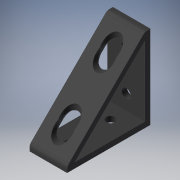
# Autodesk Inventor part: 30-4336 Aluminum
Saved by Autodesk Inventor 2019 (Build 230136000, 136)
## iProperties
Created: 2023-03-27
Part Number: 30-4336 Aluminum
Material: Generic
Catalog Web Link: www.cadenas.de
Description: 25-4136, 40-4336, 30-4366, 45-4366, 25-4136-Black, 40-4336-Black, 30-4366-Black, 45-4366-Black-4 Hole Inside Gusset Corner Bracket
Vendor: 8020
Document SubType Name: Modeling
Designer: psAdmin
Manufacturer: 8020
Mass: 18.3783 g
Surface Area: 113.769 cm^2
Volume: 18.3783 cm^3
Density: 1 g/cm^3
Appearance: PSOLRGB-191-191-191
Category: PARTsolutions
Company: 8020
Title: 30-4336
Author: Cadenas PARTsolutions
Comments: 4 Hole Inside Gusset Corner Bracket
PSOL_IDENT_0: {$CADENAS_DATA/23d-libs/8020/metric/joining_plates/25_4136.prj},242 {VTYP=3D},{NB=30-4336},{LINA=30-
PSOL_IDENT_1: 4336},{NN=25-4136, 40-4336, 30-4366, 45-4366, 25-4136-Black, 40-4336-Black, 30-4366-Black, 45-4366-B
PSOL_IDENT_2: lack},{DATE=31.07.2020 09:21:28},{GEOMDATE=11.01.2019 21:53:00},{VERSION=},{LINEID=50},{WBVAR=},{WBN
PSOL_IDENT_3: UMERIC=}  {NB=30-4336},{LINA=30-4336},{KT=DUMMY},{PN=30-4336},{SERIES=30},{MATERIAL=Aluminum},{GRADE=
PSOL_IDENT_4: 6105-T5},{FINISH=Clear Anodize},{A=27.00},{B=60.00},{C=60.00},{D=15.00},{E=15.00},{F=6.81},{G=30.00}
PSOL_IDENT_5: ,{T=4.00},{W=.049},{C1=45.000},{C2=15.000},{C3=12.700},{D1=4.000},{COLOR=.75,.75,.75}
NB: 30-4336
NN: 25-4136, 40-4336, 30-4366, 45-4366, 25-4136-Black, 40-4336-Black, 30-4366-Black, 45-4366-Black
NT: 4 Hole Inside Gusset Corner Bracket
NBSYN: $PN.
LINA: 30-4336
CATALOG: 80/20
PN: 30-4336
SERIES: 30
MATERIAL: Aluminum
GRADE: 6105-T5
FINISH: Clear Anodize
A: 27
B: 60
C: 60
D: 15
E: 15
F: 6.81
G: 30
T: 4
W: .049
SUPPLIER: 8020
ARTICLENO: 30-4336
BOMINFO: 30-4336
CREATOR: CADENAS GmbH
Autodesk Inventor part; units mm, degrees
ref_plane "YZ Plane" through (0, 0, 0) normal (1, 0, 0) x (0, 1, 0)
ref_plane "XZ Plane" through (0, 0, 0) normal (0, 1, 0) x (-1, 0, 0)
ref_plane "XY Plane" through (0, 0, 0) normal (0, 0, 1) x (1, 0, 0)
sketch "Sketch_1" plane through (0, 0, 0) normal (1, 0, 0) x (0, 1, 0)
  line L0 (2.3431, 60) -> (0, 60)
  line L1 (0, 60) -> (0, 0)
  line L2 (0, 0) -> (60, 0)
  line L3 (60, 0) -> (60, 2.3431)
  arc A0 (60, 2.3431) -> (58.8284, 5.1716) centre (56, 2.3431) ccw
  line L4 (58.8284, 5.1716) -> (5.1716, 58.8284)
  arc A1 (5.1716, 58.8284) -> (2.3431, 60) centre (2.3431, 56) ccw
  line L5 (4, 54.3431) -> (4, 4)
  line L6 (4, 4) -> (54.3431, 4)
  line L7 (54.3431, 4) -> (4, 54.3431)
  constraints: 16 end point, 4 point on circle, 2 centre point
extrude "Extrusion1" add sketch "Sketch_1" along normal mid plane 27
sketch "Sketch2" plane through (-13.5, 0, 0) normal (0, -1, 0) x (1, 0, 0)
  point P0 (13.5, 15)
hole "Hole1" at (0, 0, 15) direction (0, 1, 0) diameter 6.81 depth 4
sketch "Sketch3" plane through (13.5, 60, 0) normal (0, 0, -1) x (-1, 0, 0)
  point P0 (13.5, -45)
hole "Hole2" at (0, 15, 0) direction (0, 0, 1) diameter 6.81 depth 4
sketch "Sketch_4" plane through (0, 0, 60) normal (0, 0, 1) x (1, 0, 0)
  circle A0 centre (0, 15) radius 6.35
  constraints: 1 centre point
extrude "Extrusion2" cut sketch "Sketch_4" against normal blind 56
sketch "Sketch_5" plane through (0, 60, 0) normal (0, 1, 0) x (1, 0, 0)
  circle A0 centre (0, -15) radius 6.35
  constraints: 1 centre point
extrude "Extrusion3" cut sketch "Sketch_5" against normal blind 56
sketch "Sketch6" plane through (13.5, 60, 0) normal (0, 0, -1) x (-1, 0, 0)
  point P0 (13.5, -15)
hole "Hole3" at (0, 45, 0) direction (0, 0, 1) diameter 6.81 depth 4
sketch "Sketch7" plane through (-13.5, 0, 0) normal (0, -1, 0) x (1, 0, 0)
  point P0 (13.5, 45)
hole "Hole4" at (0, 0, 45) direction (0, 1, 0) diameter 6.81 depth 4
sketch "Sketch_8" plane through (0, 0, 60) normal (0, 0, 1) x (1, 0, 0)
  circle A0 centre (0, 45) radius 6.35
  constraints: 1 centre point
extrude "Extrusion4" cut sketch "Sketch_8" against normal blind 56
sketch "Sketch_9" plane through (0, 60, 0) normal (0, 1, 0) x (1, 0, 0)
  circle A0 centre (0, -45) radius 6.35
  constraints: 1 centre point
extrude "Extrusion5" cut sketch "Sketch_9" against normal blind 56
body "Solid1"
